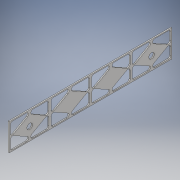
# Autodesk Inventor part: R-SideV1
Saved by Autodesk Inventor 2019 (Build 230136000, 136)
## iProperties
Created: 2021-09-15
Part Number: R-SideV1
Material: Generic
Document SubType Name: Modeling
Designer: timmy
Density: 1 g/cm^3
Appearance: Default
Author: timmy
Autodesk Inventor part; units mm, degrees
ref_plane "YZ Plane" through (0, 0, 0) normal (1, 0, 0) x (0, 1, 0)
ref_plane "XZ Plane" through (0, 0, 0) normal (0, 1, 0) x (-1, 0, 0)
ref_plane "XY Plane" through (0, 0, 0) normal (0, 0, 1) x (1, 0, 0)
sketch "Sketch1" plane through (0, 0, 0) normal (1, 0, 0) x (0, 1, 0)
  line L0 (0, 0) -> (152.4, 0)
  line L1 (152.4, 0) -> (152.4, -914.4)
  line L2 (152.4, -914.4) -> (0, -914.4)
  line L3 (0, -914.4) -> (0, 0)
  dimension "d0" = 152.4
  dimension "d1" = 914.4
  constraints: 8 end point, 2 parallel, 1 horizontal, 1 perpendicular
  measures "d0" distance of L1.end L2.end
  measures "d1" distance of L0.end L1.end
extrude "Extrusion1" add sketch "Sketch1" along normal blind 6.35
sketch "Sketch2" plane through (6.35, 0, 0) normal (1, 0, 0) x (0, 0, -1)
  line L0 (0, 152.4) -> (0, 0) construction
  line L1 (914.4, 152.4) -> (0, 152.4) construction
  line L2 (0, 152.4) -> (457.2, 152.4) construction
  line L3 (228.6, 152.4) -> (0, 152.4) construction
  line L4 (17.9147, 146.1725) -> (95.9969, 146.1725)
  arc A0 (101.8461, 123.5552) -> (95.9969, 146.1725) centre (95.9969, 134.1075) ccw
  line L5 (101.8461, 123.5552) -> (23.7639, 80.2737)
  arc A1 (5.8497, 90.826) -> (23.7639, 80.2737) centre (17.9147, 90.826) ccw
  line L6 (5.8497, 90.826) -> (5.8497, 134.1075)
  arc A2 (17.9147, 146.1725) -> (5.8497, 134.1075) centre (17.9147, 134.1075) ccw
  line L7 (210.6853, 146.1725) -> (132.6031, 146.1725)
  arc A3 (132.6031, 146.1725) -> (126.7539, 123.5552) centre (132.6031, 134.1075) ccw
  line L8 (126.7539, 123.5552) -> (204.8361, 80.2737)
  arc A4 (204.8361, 80.2737) -> (222.7503, 90.826) centre (210.6853, 90.826) ccw
  line L9 (222.7503, 90.826) -> (222.7503, 134.1075)
  arc A5 (222.7503, 134.1075) -> (210.6853, 146.1725) centre (210.6853, 134.1075) ccw
  line L10 (17.9147, 6.2275) -> (95.9969, 6.2275)
  arc A6 (95.9969, 6.2275) -> (101.8461, 28.8448) centre (95.9969, 18.2925) ccw
  line L11 (101.8461, 28.8448) -> (23.7639, 72.1263)
  arc A7 (23.7639, 72.1263) -> (5.8497, 61.574) centre (17.9147, 61.574) ccw
  line L12 (5.8497, 61.574) -> (5.8497, 18.2925)
  arc A8 (5.8497, 18.2925) -> (17.9147, 6.2275) centre (17.9147, 18.2925) ccw
  line L13 (126.7539, 28.8448) -> (204.8361, 72.1263)
  line L14 (210.6853, 6.2275) -> (132.6031, 6.2275)
  line L15 (222.7503, 61.574) -> (222.7503, 18.2925)
  arc A9 (222.7503, 61.574) -> (204.8361, 72.1263) centre (210.6853, 61.574) ccw
  arc A10 (210.6853, 6.2275) -> (222.7503, 18.2925) centre (210.6853, 18.2925) ccw
  arc A11 (126.7539, 28.8448) -> (132.6031, 6.2275) centre (132.6031, 18.2925) ccw
  line L16 (439.2853, 146.1725) -> (361.2031, 146.1725)
  arc A12 (361.2031, 146.1725) -> (355.3539, 123.5552) centre (361.2031, 134.1075) ccw
  line L17 (355.3539, 123.5552) -> (433.4361, 80.2737)
  arc A13 (433.4361, 80.2737) -> (451.3503, 90.826) centre (439.2853, 90.826) ccw
  line L18 (451.3503, 90.826) -> (451.3503, 134.1075)
  arc A14 (451.3503, 134.1075) -> (439.2853, 146.1725) centre (439.2853, 134.1075) ccw
  line L19 (330.4461, 123.5552) -> (252.3639, 80.2737)
  line L20 (246.5147, 146.1725) -> (324.5969, 146.1725)
  line L21 (234.4497, 90.826) -> (234.4497, 134.1075)
  arc A15 (234.4497, 90.826) -> (252.3639, 80.2737) centre (246.5147, 90.826) ccw
  arc A16 (246.5147, 146.1725) -> (234.4497, 134.1075) centre (246.5147, 134.1075) ccw
  arc A17 (330.4461, 123.5552) -> (324.5969, 146.1725) centre (324.5969, 134.1075) ccw
  arc A18 (439.2853, 6.2275) -> (451.3503, 18.2925) centre (439.2853, 18.2925) ccw
  line L22 (439.2853, 6.2275) -> (361.2031, 6.2275)
  line L23 (355.3539, 28.8448) -> (433.4361, 72.1263)
  arc A19 (355.3539, 28.8448) -> (361.2031, 6.2275) centre (361.2031, 18.2925) ccw
  line L24 (451.3503, 61.574) -> (451.3503, 18.2925)
  arc A20 (451.3503, 61.574) -> (433.4361, 72.1263) centre (439.2853, 61.574) ccw
  arc A21 (324.5969, 6.2275) -> (330.4461, 28.8448) centre (324.5969, 18.2925) ccw
  line L25 (246.5147, 6.2275) -> (324.5969, 6.2275)
  arc A22 (252.3639, 72.1263) -> (234.4497, 61.574) centre (246.5147, 61.574) ccw
  line L26 (234.4497, 61.574) -> (234.4497, 18.2925)
  arc A23 (234.4497, 18.2925) -> (246.5147, 6.2275) centre (246.5147, 18.2925) ccw
  line L27 (330.4461, 28.8448) -> (252.3639, 72.1263)
  line L28 (896.5064, 147.907) -> (818.4249, 147.5987)
  arc A24 (818.4249, 147.5987) -> (812.6651, 124.9585) centre (818.4726, 135.5338) ccw
  line L29 (812.6651, 124.9585) -> (890.9175, 81.9857)
  arc A25 (890.9175, 81.9857) -> (908.7899, 92.6086) centre (896.725, 92.561) ccw
  line L30 (908.7899, 92.6086) -> (908.619, 135.8897)
  arc A26 (908.619, 135.8897) -> (896.5064, 147.907) centre (896.5541, 135.8421) ccw
  line L31 (787.7574, 124.8602) -> (709.8468, 81.2707)
  line L32 (703.7374, 147.1459) -> (781.8189, 147.4542)
  line L33 (691.891, 91.7522) -> (691.7201, 135.0333)
  arc A27 (691.891, 91.7522) -> (709.8468, 81.2707) centre (703.9559, 91.7998) ccw
  arc A28 (703.7374, 147.1459) -> (691.7201, 135.0333) centre (703.785, 135.081) ccw
  arc A29 (787.7574, 124.8602) -> (781.8189, 147.4542) centre (781.8665, 135.3893) ccw
  arc A30 (897.059, 7.9631) -> (909.0763, 20.0757) centre (897.0113, 20.028) ccw
  line L34 (897.059, 7.9631) -> (818.9775, 7.6548)
  line L35 (813.039, 30.2488) -> (890.9496, 73.8383)
  arc A31 (813.039, 30.2488) -> (818.9775, 7.6548) centre (818.9298, 19.7197) ccw
  line L36 (908.9054, 63.3568) -> (909.0763, 20.0757)
  arc A32 (908.9054, 63.3568) -> (890.9496, 73.8383) centre (896.8405, 63.3092) ccw
  arc A33 (782.3715, 7.5103) -> (788.1313, 30.1505) centre (782.3238, 19.5752) ccw
  line L37 (704.29, 7.202) -> (782.3715, 7.5103)
  arc A34 (709.8789, 73.1233) -> (692.0065, 62.5004) centre (704.0714, 62.548) ccw
  line L38 (692.0065, 62.5004) -> (692.1774, 19.2192)
  arc A35 (692.1774, 19.2192) -> (704.29, 7.202) centre (704.2423, 19.2669) ccw
  line L39 (788.1313, 30.1505) -> (709.8789, 73.1233)
  arc A36 (463.2928, 90.8496) -> (481.2485, 80.3681) centre (475.3577, 90.8972) ccw
  line L40 (463.2928, 90.8496) -> (463.1219, 134.1307)
  line L41 (559.1592, 123.9576) -> (481.2485, 80.3681)
  arc A37 (559.1592, 123.9576) -> (553.2207, 146.5516) centre (553.2683, 134.4867) ccw
  line L42 (475.1392, 146.2433) -> (553.2207, 146.5516)
  arc A38 (475.1392, 146.2433) -> (463.1219, 134.1307) centre (475.1868, 134.1784) ccw
  arc A39 (680.3071, 62.4542) -> (662.3514, 72.9357) centre (668.2422, 62.4066) ccw
  line L43 (680.3071, 62.4542) -> (680.478, 19.1731)
  arc A40 (668.4608, 7.0605) -> (680.478, 19.1731) centre (668.4131, 19.1254) ccw
  line L44 (584.4408, 29.3462) -> (662.3514, 72.9357)
  arc A41 (584.4408, 29.3462) -> (590.3793, 6.7522) centre (590.3316, 18.8171) ccw
  arc A42 (662.3192, 81.0831) -> (680.1916, 91.706) centre (668.1267, 91.6584) ccw
  arc A43 (481.2807, 72.2207) -> (463.4083, 61.5978) centre (475.4732, 61.6454) ccw
  line L45 (559.5331, 29.2479) -> (481.2807, 72.2207)
  arc A44 (553.7733, 6.6077) -> (559.5331, 29.2479) centre (553.7256, 18.6726) ccw
  line L46 (463.4083, 61.5978) -> (463.5792, 18.3166)
  arc A45 (463.5792, 18.3166) -> (475.6917, 6.2994) centre (475.6441, 18.3643) ccw
  line L47 (584.0668, 124.0559) -> (662.3192, 81.0831)
  line L48 (667.9082, 147.0044) -> (589.8267, 146.6961)
  arc A46 (589.8267, 146.6961) -> (584.0668, 124.0559) centre (589.8743, 134.6312) ccw
  line L49 (680.1916, 91.706) -> (680.0208, 134.9871)
  arc A47 (680.0208, 134.9871) -> (667.9082, 147.0044) centre (667.9558, 134.9395) ccw
  line L50 (475.6917, 6.2994) -> (553.7733, 6.6077)
  line L51 (668.4608, 7.0605) -> (590.3793, 6.7522)
  circle A48 centre (114.3, 72.0167) radius 15.5575
  circle A49 centre (800.4147, 73.3712) radius 15.5575
  constraints: 100 end point, 96 point on circle, 50 centre point, 2 midpoint, 1 collinear, 1 perpendicular
extrude "Extrusion2" cut sketch "Sketch2" against normal blind 6.35
body "Solid1"
